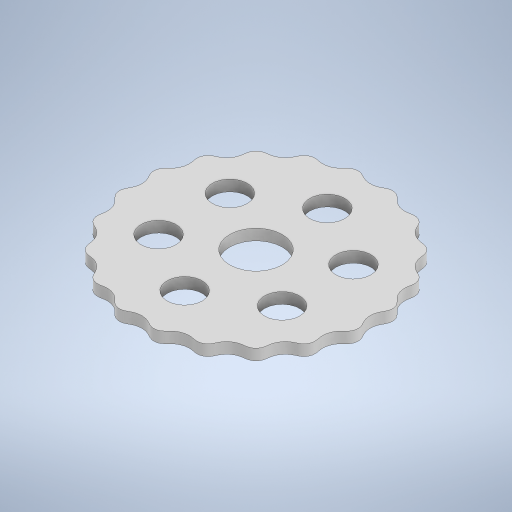
# Autodesk Inventor part: Epitrochoid
Saved by Autodesk Inventor 2023 (Build 270158000, 158)
## iProperties
Created: 2023-01-17
Part Number: Epitrochoid
Material: Generic
Document SubType Name: Modeling
Designer: caden
Density: 1 g/cm^3
Appearance: Default
Author: caden
Autodesk Inventor part; units mm, degrees
ref_plane "YZ Plane" through (0, 0, 0) normal (1, 0, 0) x (0, 1, 0)
ref_plane "XZ Plane" through (0, 0, 0) normal (0, 1, 0) x (-1, 0, 0)
ref_plane "XY Plane" through (0, 0, 0) normal (0, 0, 1) x (1, 0, 0)
sketch "Sketch2" plane through (0, 0, 0) normal (0, 1, 0) x (-1, 0, 0)
  spline S0 degree 5 poles (52, 0) (51.9971, -1.2607) (52.2669, -2.5082) (52.7194, -3.7477) (53.9313, -5.1861) (54.3906, -7.0888) (54.4411, -7.6616) (54.3551, -8.9458) (53.9203, -10.0362) (53.6379, -10.5866) (52.1566, -12.3389) (50.3896, -13.4773) (49.4928, -15.3337) (48.8918, -17.51) (49.1349, -20.2532) (49.3828, -21.0243) (49.7232, -22.5528) (49.4072, -24.1021) (49.2179, -24.6637) (48.59, -25.8082) (47.7243, -26.6329) (47.2332, -26.9969) (44.993, -28.0598) (42.9159, -29.0048) (41.4975, -30.8139) (40.6824, -32.9781) (40.393, -35.6037) (40.3684, -36.2297) (39.9658, -37.559) (39.2202, -38.6234) (38.7461, -39.1136) (37.7292, -39.8726) (36.4551, -40.316) (35.8527, -40.3747) (33.2595, -40.6301) (31.0353, -41.3331) (29.1967, -42.724) (28.124, -44.7764) (27.0879, -47.0696) (26.7578, -47.5734) (25.9327, -48.4916) (24.8259, -49.1453) (24.2456, -49.3656) (22.8, -49.7003) (21.318, -49.4645) (20.6191, -49.2204) (17.9097, -48.8633) (15.7047, -49.3102) (13.706, -50.1891) (12.4718, -51.9548) (10.7262, -53.5444) (10.1816, -53.8459) (9.119, -54.3129) (7.8176, -54.4466) (7.2501, -54.4082) (5.439, -54.0466) (4.027, -52.9365) (3.0169, -52.4579) (0.4434, -51.7489) (-1.9852, -52.0959) (-3.4655, -52.5149) (-4.9442, -53.7984) (-6.9249, -54.3689) (-7.511, -54.4299) (-8.7641, -54.3928) (-9.8959, -53.9884) (-10.4442, -53.7245) (-12.1913, -52.3637) (-13.2584, -50.6143) (-14.9196, -49.7179) (-17.0895, -48.9439) (-19.8381, -49.0541) (-20.7102, -49.2829) (-22.2954, -49.7348) (-23.9535, -49.4464) (-24.5036, -49.2825) (-25.6786, -48.686) (-26.5101, -47.8642) (-26.9031, -47.3857) (-28.0034, -45.2088) (-28.8187, -43.1262) (-30.5816, -41.6837) (-32.6708, -40.7596) (-35.3262, -40.4092) (-35.9869, -40.4113) (-37.3715, -40.0635) (-38.5032, -39.3175) (-38.9972, -38.8712) (-39.7839, -37.8838) (-40.2558, -36.6666) (-40.3526, -36.0777) (-40.5992, -33.5186) (-41.1837, -31.2542) (-42.5474, -29.3937) (-44.5551, -28.2015) (-46.8918, -27.1774) (-47.411, -26.8831) (-48.3877, -26.0566) (-49.0667, -24.9863) (-49.3202, -24.3867) (-49.6702, -23.0343) (-49.5267, -21.5903) (-49.3034, -20.942) (-48.8559, -18.2798) (-49.1641, -16.0328) (-50.0121, -13.9429) (-51.7597, -12.5942) (-53.4428, -10.8641) (-53.7646, -10.3318) (-54.2665, -9.285) (-54.446, -7.9787) (-54.4219, -7.4104) (-54.1431, -5.6913) (-53.1521, -4.3088) (-52.6642, -3.4729) (-51.7928, -0.8825) (-51.9584, 1.4605) (-52.3292, 3.1894) (-53.6543, 4.7123) (-54.3414, 6.7626) (-54.4147, 7.36) (-54.424, 8.5801) (-54.052, 9.757) (-53.8043, 10.2997) (-52.5734, 12.0256) (-50.8626, 13.0494) (-49.9871, 14.4732) (-49.0219, 16.66) (-48.9869, 19.3706) (-49.1695, 20.3809) (-49.731, 22.03) (-49.484, 23.7995) (-49.3379, 24.3479) (-48.7815, 25.5406) (-47.9937, 26.3904) (-47.5294, 26.8057) (-45.4284, 27.949) (-43.3564, 28.6412) (-41.9012, 30.3297) (-40.8644, 32.336) (-40.4269, 35.015) (-40.4431, 35.7227) (-40.1642, 37.1671) (-39.4074, 38.3838) (-38.9967, 38.8725) (-38.0261, 39.6979) (-36.8661, 40.1894) (-36.2835, 40.3255) (-33.7605, 40.5856) (-31.4777, 41.0454) (-29.5976, 42.3815) (-28.2978, 44.325) (-27.267, 46.6965) (-27.0071, 47.2363) (-26.1847, 48.2747) (-25.1406, 48.9848) (-24.529, 49.269) (-23.2527, 49.6363) (-21.8437, 49.5704) (-21.2288, 49.3792) (-18.6156, 48.8676) (-16.3261, 49.0461) (-14.184, 49.8575) (-12.7132, 51.5697) (-11.0007, 53.3325) (-10.4884, 53.6748) (-9.4421, 54.2171) (-8.147, 54.4383) (-7.5665, 54.4324) (-5.942, 54.2212) (-4.5837, 53.3556) (-3.8741, 52.8728) (-1.31, 51.8615) (0.9685, 51.8542) (2.9131, 52.168) (4.4971, 53.5041) (6.6007, 54.3073) (7.2071, 54.3955) (8.3956, 54.4483) (9.6176, 54.1115) (10.1528, 53.8784) (11.8431, 52.7796) (12.8465, 51.1328) (14.0171, 50.2941) (16.2314, 49.1275) (18.8553, 48.9425) (20.0457, 49.0505) (21.7584, 49.7092) (23.6413, 49.5195) (24.1968, 49.3847) (25.3931, 48.8766) (26.274, 48.1137) (26.7041, 47.6656) (27.8903, 45.6554) (28.4763, 43.6066) (30.0508, 42.1607) (31.9761, 40.9983) (34.6652, 40.4514) (35.4334, 40.463) (36.9473, 40.2646) (38.2624, 39.4926) (38.7423, 39.1193) (39.6117, 38.1604) (40.1189, 37.0546) (40.2929, 36.4742) (40.5855, 33.9905) (40.9166, 31.7115) (42.2212, 29.8128) (44.0823, 28.4182) (46.4796, 27.3589) (47.0475, 27.1286) (48.1497, 26.3204) (48.9013, 25.2859) (49.2104, 24.6754) (49.6007, 23.4537) (49.5982, 22.0814) (49.4449, 21.4858) (48.8965, 18.9168) (48.9482, 16.5972) (49.7256, 14.4221) (51.3801, 12.8406) (53.2138, 11.134) (53.5714, 10.6587) (54.1707, 9.579) (54.4183, 8.3334) (54.4448, 7.7131) (54.271, 6.1819) (53.5583, 4.8694) (53.0321, 4.1716) (52.7094, 3.3781) (52.4269, 2.5736) knots 0 0 0 0 0 0 0.017503 0.017503 0.017503 0.026054 0.026054 0.026054 0.034326 0.034326 0.034326 0.056974 0.056974 0.056974 0.069321 0.069321 0.069321 0.078137 0.078137 0.078137 0.08638 0.08638 0.08638 0.111809 0.111809 0.111809 0.121218 0.121218 0.121218 0.130155 0.130155 0.130155 0.139119 0.139119 0.139119 0.164872 0.164872 0.164872 0.173212 0.173212 0.173212 0.182079 0.182079 0.182079 0.193361 0.193361 0.193361 0.217058 0.217058 0.217058 0.225281 0.225281 0.225281 0.233915 0.233915 0.233915 0.249825 0.249825 0.249825 0.26892 0.26892 0.26892 0.277386 0.277386 0.277386 0.285726 0.285726 0.285726 0.307122 0.307122 0.307122 0.320728 0.320728 0.320728 0.329481 0.329481 0.329481 0.337684 0.337684 0.337684 0.362598 0.362598 0.362598 0.372599 0.372599 0.372599 0.381521 0.381521 0.381521 0.390164 0.390164 0.390164 0.416058 0.416058 0.416058 0.424567 0.424567 0.424567 0.433473 0.433473 0.433473 0.443883 0.443883 0.443883 0.468418 0.468418 0.468418 0.476618 0.476618 0.476618 0.485329 0.485329 0.485329 0.49973 0.49973 0.49973 0.520334 0.520334 0.520334 0.528718 0.528718 0.528718 0.537136 0.537136 0.537136 0.557106 0.557106 0.557106 0.57214 0.57214 0.57214 0.58082 0.58082 0.58082 0.589026 0.589026 0.589026 0.613223 0.613223 0.613223 0.623988 0.623988 0.623988 0.63288 0.63288 0.63288 0.641305 0.641305 0.641305 0.667161 0.667161 0.667161 0.675929 0.675929 0.675929 0.684858 0.684858 0.684858 0.694581 0.694581 0.694581 0.719745 0.719745 0.719745 0.727959 0.727959 0.727959 0.736739 0.736739 0.736739 0.749775 0.749775 0.749775 0.771741 0.771741 0.771741 0.78005 0.78005 0.78005 0.788552 0.788552 0.788552 0.806975 0.806975 0.806975 0.823557 0.823557 0.823557 0.832156 0.832156 0.832156 0.840397 0.840397 0.840397 0.863667 0.863667 0.863667 0.875384 0.875384 0.875384 0.884232 0.884232 0.884232 0.892521 0.892521 0.892521 0.918159 0.918159 0.918159 0.927298 0.927298 0.927298 0.936236 0.936236 0.936236 0.945433 0.945433 0.945433 0.971029 0.971029 0.971029 0.979305 0.979305 0.979305 0.988144 0.988144 0.988144 1 1 1 1 1 1
  arc A0 (52.4269, 2.5736) -> (52, 0) centre (59.9711, 0) ccw
  point P0 (0, 0)
  constraints: 2 point on circle, 1 centre point, 4 other
extrude "Extrusion2" add sketch "Sketch2" along normal blind 5
sketch "Sketch3" plane through (0, 5, 0) normal (0, 1, 0) x (1, 0, 0)
  circle A0 centre (0, 0) radius 12
  circle A1 centre (0, 0) radius 32.5 construction
  circle A2 centre (0, 32.5) radius 8
  circle A3 centre (-28.1458, 16.25) radius 8
  circle A4 centre (-28.1458, -16.25) radius 8
  circle A5 centre (0, -32.5) radius 8
  circle A6 centre (28.1458, -16.25) radius 8
  circle A7 centre (28.1458, 16.25) radius 8
  circle A8 centre (0, 32.5) radius 7.25 construction
  circle A9 centre (0, 32.5) radius 11 construction
  dimension "d12" = 65
  dimension "d10" = 24
  dimension "d11" = 16
  dimension "d15" = 360
  dimension "d20" = 14.5
  dimension "d21" = 22
  constraints: 9 centre point, 4 coincident, 1 vertical alignment, 15 other
  measures "d10" diameter of A0
  measures "d11" diameter of A2
  measures "d20" diameter of A8
  measures "d21" diameter of A9
extrude "Extrusion3" cut sketch "Sketch3" against normal through all
equation "curve S0 of \"Sketch2\": x = (60*cos(t))-(6.5*cos(t+atan(sin((1-21)*t)/((60/(1.5*21))-cos((1-21)*t)))))-(1.5*cos(21*t)); y = (-60*sin(t))+(6.5*sin(t+atan(sin((1-21)*t)/((60/(1.5*21))-cos((1-21)*t)))))+("
body "Solid2"
